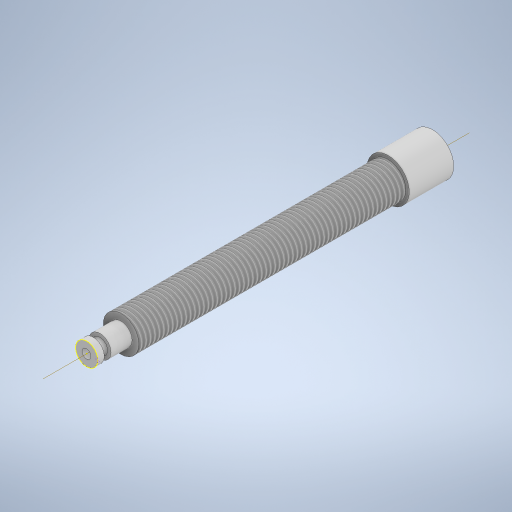
# Autodesk Inventor part: Trapezspindle
Saved by Autodesk Inventor 2023 (Build 270158000, 158)
## iProperties
Created: 2023-05-10
Part Number: Trapezspindle
Material: Generic
Document SubType Name: Modeling
Designer: dell
Density: 1 g/cm^3
Appearance: Default
Author: dell
Autodesk Inventor part; units mm, degrees
ref_plane "YZ Plane" through (0, 0, 0) normal (1, 0, 0) x (0, 1, 0)
ref_plane "XZ Plane" through (0, 0, 0) normal (0, 1, 0) x (-1, 0, 0)
sketch "Sketch1" plane through (0, 0, 0) normal (0, 0, 1) x (1, 0, 0)
  circle A0 centre (0, 0) radius 8
  dimension "d0" = 16
  constraints: 1 centre point, 1 coincident
  measures "d0" diameter of A0
extrude "Extrusion1" add sketch "Sketch1" along normal blind 120
sketch "Sketch2" plane through (0, 0, 120) normal (0, 0, 1) x (1, 0, 0)
  circle A0 centre (0, 0) radius 5
  dimension "d3" = 10
  constraints: 1 centre point, 1 coincident
  measures "d3" diameter of A0
extrude "Extrusion2" add sketch "Sketch2" along normal blind 9.5
sketch "Sketch5" plane through (0, 0, 129.5) normal (0, 0, 1) x (1, 0, 0)
  circle A0 centre (0, 0) radius 5
  constraints: 1 centre point, 1 coincident
extrude "Extrusion4" add sketch "Sketch5" along normal blind 6
sketch "Sketch8" plane through (0, 0, 135.5) normal (0, 0, 1) x (1, 0, 0)
  circle A0 centre (0, 0) radius 5 projected
  circle A1 centre (0, 0) radius 2
  dimension "d27" = 4
  constraints: 1 centre point, 1 coincident
  measures "d27" diameter of A1
extrude "Extrusion7" cut sketch "Sketch8" against normal blind 189 contours A1
sketch "Sketch10" plane through (0, 0, 0) normal (0, 0, -1) x (-1, 0, 0)
  circle A0 centre (0, 0) radius 2 projected
  circle A1 centre (0, 0) radius 9.5
  dimension "d44" = 19
  constraints: 1 centre point, 1 coincident
  measures "d44" diameter of A1
extrude "Extrusion9" add sketch "Sketch10" along normal blind 20 contours A0 | A1
sketch "Sketch11" plane through (0, 0, -20) normal (0, 0, -1) x (-1, 0, 0)
  circle A0 centre (0, 0) radius 2 projected
  circle A1 centre (0, 0) radius 2
  constraints: 1 centre point, 1 coincident
extrude "Extrusion10" cut sketch "Sketch11" against normal blind 20
sketch "Sketch12" plane through (0, 0, 135.5) normal (0, 0, 1) x (1, 0, 0)
  circle A0 centre (0, 0) radius 5 projected
  point P0 (5, 0)
  constraints: 1 horizontal alignment, 1 other
ref_plane "Work Plane1" through (5, 0, 135.5) normal (0, 1, 0) x (-1, 0, 0)
sketch "Sketch14" plane through (5, 0, 135.5) normal (0, 1, 0) x (-1, 0, 0)
  point P0 (5, -135.5)
sketch "Sketch15" plane through (5, 0, 135.5) normal (0, 1, 0) x (-1, 0, 0)
  arc A0 (8.5, -3) -> (8.5, -6) centre (8.5, -4.5) ccw
  line L0 (13, -15.5) -> (-3, -15.5) projected
  line L1 (5, -186.6) -> (5, 31.1) projected
  line L2 (8.5, -6) -> (10, -6)
  line L3 (8.5, -3) -> (10, -3)
  line L4 (10, -15.5) -> (10, 0) projected
  line L5 (10, -3) -> (10, -6)
  point P0 (5, -135.5)
  point P1 (10, -6)
  dimension "d67" = 3
  dimension "d68" = 11
  dimension "d69" = 3.5
  constraints: 6 end point, 2 horizontal, 2 point on circle, 1 centre point, 1 collinear, 1 point on line, 1 tangent
  measures "d67" diameter of A0
  measures "d68" distance from line of L0 A0.centre
  measures "d69" distance from line of L1 A0.centre
revolve "Revolution2" cut sketch "Sketch15" angle 360 about axis through (0, 0, 120) along (0, 0, -1)
thread "Thread1" size "M16x2" class "6g" standard "ANSI Metric M Profile" full length
body "Solid1"
